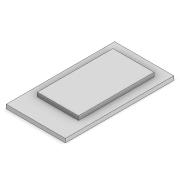
# Autodesk Inventor part: Gyro
Saved by Autodesk Inventor 2020 (Build 240168000, 168)
## iProperties
Created: 2019-08-08
Part Number: Gyro
Material: Generic
Document SubType Name: Modeling
Designer: chitl
Density: 1 g/cm^3
Appearance: Default
Author: chitl
Autodesk Inventor part; units mm, degrees
ref_plane "YZ Plane" through (0, 0, 0) normal (1, 0, 0) x (0, 1, 0)
ref_plane "XZ Plane" through (0, 0, 0) normal (0, 1, 0) x (-1, 0, 0)
ref_plane "XY Plane" through (0, 0, 0) normal (0, 0, 1) x (1, 0, 0)
sketch "Sketch1" plane through (0, 0, 0) normal (0, 1, 0) x (-1, 0, 0)
  line L0 (0, 0) -> (-24, 0)
  line L1 (-24, 0) -> (-24, 44)
  line L2 (-24, 44) -> (0, 44)
  line L3 (0, 44) -> (0, 0)
  dimension "d0" = 24
  dimension "d1" = 44
  constraints: 8 end point, 2 parallel, 1 horizontal, 1 perpendicular
  measures "d0" distance of L1.end L2.end
  measures "d1" distance of L0.end L1.end
extrude "Extrusion1" add sketch "Sketch1" along normal blind 1.6
sketch "Sketch3" plane through (0, 1.6, 0) normal (0, 1, 0) x (1, 0, 0)
  line L0 (3.6828, -4.4062) -> (20.3867, -4.4062)
  line L1 (20.3867, -4.4062) -> (20.3867, -35.052)
  line L2 (20.3867, -35.052) -> (3.6828, -35.052)
  line L3 (3.6828, -35.052) -> (3.6828, -4.4062)
  line L4 (4.8665, -37.9456) -> (18.6769, -37.9456)
  line L5 (18.6769, -37.9456) -> (18.6769, -41.7599)
  line L6 (18.6769, -41.7599) -> (4.8665, -41.7599)
  line L7 (4.8665, -41.7599) -> (4.8665, -37.9456)
  point P0 (0, 0)
  constraints: 16 end point, 4 parallel, 2 horizontal, 2 perpendicular
extrude "Extrusion3" add sketch "Sketch3" along normal blind 1.6 contours L0 L1 L2 L3
sketch "Sketch4" plane through (0, 1.6, 0) normal (0, 1, 0) x (1, 0, 0)
  point P0 (0, 0)
body "Solid1"
